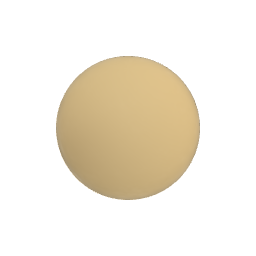
Scene (Autodesk Fusion 360 archive; units mm, degrees)
design "ball"
Autodesk Fusion 360 part; units mm, degrees
sphere "PrimitivaSfera1" add diameter 200 placed x (1, 0, 0) y (0, 1, 0) z (0, 0, 1) at (0, 0, 0)
component "Component" placed x (1, 0, 0) y (0, 1, 0) z (0, 0, 1) at (0, 0, 0)

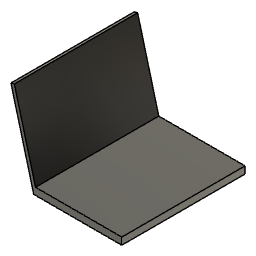
design "laptop"
Autodesk Fusion 360 part; units mm, degrees
sketch "Schizzo1" plane through (0, 0, 0) normal (0, 1, 0) x (1, 0, 0)
  line L0 (0, 0) -> (-64.7048, -241.4815)
  line L1 (-64.7048, -241.4815) -> (-55.0455, -244.0696)
  line L2 (-55.0455, -244.0696) -> (4.9938, -20)
  line L3 (4.9938, -20) -> (250, -20)
  line L4 (250, -20) -> (250, 0)
  line L5 (250, 0) -> (0, 0)
  dimension "d1" = 75
  dimension "d2" = 250
  dimension "d3" = 250
  dimension "d4" = 20
  dimension "d5" = 10
  constraint coincident L0.start L5.end
  constraint perpendicular L0 L1
  constraint perpendicular L1 L2
  constraint horizontal L3
  constraint perpendicular L3 L4
  constraint horizontal L5
  measures "d1" angle of L0 L5
  measures "d2" distance of L0.start L4.end
  measures "d3" distance of L0.start L0.end
  measures "d4" distance of L3.end L4.end
  measures "d5" distance of L0.end L1.end
extrude "Estrusione1" add sketch "Schizzo1" along normal blind 350
component "Component" placed x (1, 0, 0) y (0, 1, 0) z (0, 0, 1) at (0, 0, 0)

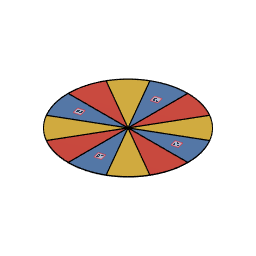
design "paracadute"
Autodesk Fusion 360 part; units mm, degrees
sketch "Schizzo1" plane through (0, 0, 0) normal (0, 0, 1) x (1, 0, 0)
  circle A0 centre (0, 0) radius 1500
  line L0 (0, 0) -> (0, 1500)
  line L1 (0, 0) -> (-750, 1299.0381)
  line L2 (0, 0) -> (-1299.0381, 750)
  line L3 (0, 0) -> (-1500, 0)
  line L4 (0, 0) -> (-1299.0381, -750)
  line L5 (0, 0) -> (-750, -1299.0381)
  line L6 (0, 0) -> (0, -1500)
  line L7 (0, 0) -> (750, -1299.0381)
  line L8 (0, 0) -> (1299.0381, -750)
  line L9 (0, 0) -> (1500, 0)
  line L10 (0, 0) -> (1299.0381, 750)
  line L11 (0, 0) -> (750, 1299.0381)
  dimension "d1" = 3000
  dimension "d3" = 360
  constraint coincident A0.centre L0.start
  constraint coincident A0 L0.end
  constraint vertical L0
  measures "d1" diameter of A0
extrude "Estrusione1" add sketch "Schizzo1" along normal blind 10 contours A0 L0 L11 makes body 1
pattern_circular "Serie C1" count 12 over 360 about axis through (0, 0, 1.75) along (0, 0, 1) of bodies 1 makes body 2 at (-441.3417, 894.9525, 0) makes body 3 at (-829.6894, 554.3807, 0) makes body 4 at (-995.7224, 65.2631, 0) makes body 5 at (-894.9525, -441.3417, 0) makes body 6 at (-554.3807, -829.6894, 0) makes body 7 at (-65.2631, -995.7224, 0) makes body 8 at (441.3417, -894.9525, 0) makes body 9 at (829.6894, -554.3807, 0) makes body 10 at (995.7224, -65.2631, 0) makes body 11 at (894.9525, 441.3417, 0) makes body 12 at (554.3807, 829.6894, 0)
sketch "Schizzo2" plane through (0, 0, 10) normal (0, 0, 1) x (-1, 0, 0)
  line L0 (0, 0) -> (0, -1500)
  arc A0 (0, -1500) -> (750, -1299.0381) centre (0, 0) ccw
  line L1 (750, -1299.0381) -> (0, 0)
  line L2 (388.2286, -1448.8887) -> (0, 0) construction
  line L3 (205.786, -1057.7817) -> (350.6749, -1018.9588)
  line L4 (350.6749, -1018.9588) -> (311.8521, -874.07)
  line L5 (311.8521, -874.07) -> (166.9632, -912.8928)
  line L6 (166.9632, -912.8928) -> (205.786, -1057.7817)
  line L7 (205.786, -1057.7817) -> (311.8521, -874.07) construction
  line L8 (350.6749, -1018.9588) -> (166.9632, -912.8928) construction
  line L9 (874.07, 311.8521) -> (912.8928, 166.9632)
  line L10 (1018.9588, 350.6749) -> (874.07, 311.8521)
  line L11 (1057.7817, 205.786) -> (1018.9588, 350.6749)
  line L12 (912.8928, 166.9632) -> (1057.7817, 205.786)
  line L13 (-311.8521, 874.07) -> (-166.9632, 912.8928)
  line L14 (-350.6749, 1018.9588) -> (-311.8521, 874.07)
  line L15 (-205.786, 1057.7817) -> (-350.6749, 1018.9588)
  line L16 (-166.9632, 912.8928) -> (-205.786, 1057.7817)
  line L17 (-874.07, -311.8521) -> (-912.8928, -166.9632)
  line L18 (-1018.9588, -350.6749) -> (-874.07, -311.8521)
  line L19 (-1057.7817, -205.786) -> (-1018.9588, -350.6749)
  line L20 (-912.8928, -166.9632) -> (-1057.7817, -205.786)
  point P0 (258.819, -965.9258)
  dimension "d8" = 500
  dimension "d9" = 150
  dimension "d10" = 150
  dimension "d12" = 360
  constraint midpoint A0 L2.start
  constraint coincident L0.start A0.centre
  constraint perpendicular L3 L4
  constraint parallel L3 L5
  constraint parallel L4 L6
  constraint coincident L7 P0
  constraint coincident L8 P0
  constraint coincident L2 P0
  constraint parallel L2 L6
  measures "d8" distance of L2.start P0
  measures "d9" distance of L3.start L3.end
  measures "d10" distance of L3.start L5.end
component "Component" placed x (1, 0, 0) y (0, 1, 0) z (0, 0, 1) at (0, 0, 0)

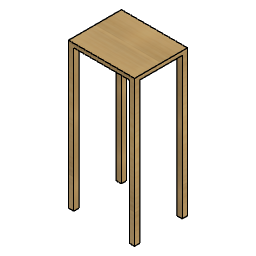
design "table"
Autodesk Fusion 360 part; units mm, degrees
box "PrimitivaParallelepipedo1" add length 400 width 500 height 30 placed x (0, 1, 0) y (-1, 0, 0) z (0, 0, 1) at (500, 0, 0)
sketch "Schizzo2" plane through (0, 0, 0) normal (0, 0, -1) x (1, 0, 0)
  line L0 (0, -400) -> (500, -400)
  line L1 (500, -400) -> (500, 0)
  line L2 (500, 0) -> (0, 0)
  line L3 (0, 0) -> (0, -400)
  line L4 (0, 0) -> (40, 0)
  line L5 (40, 0) -> (40, -40)
  line L6 (40, -40) -> (0, -40)
  line L7 (0, -40) -> (0, 0)
  line L8 (500, 0) -> (460, 0)
  line L9 (460, 0) -> (460, -40)
  line L10 (460, -40) -> (500, -40)
  line L11 (500, -40) -> (500, 0)
  line L12 (500, -400) -> (460, -400)
  line L13 (460, -400) -> (460, -360)
  line L14 (460, -360) -> (500, -360)
  line L15 (500, -360) -> (500, -400)
  line L16 (0, -400) -> (40, -400)
  line L17 (40, -400) -> (40, -360)
  line L18 (40, -360) -> (0, -360)
  line L19 (0, -360) -> (0, -400)
  dimension "d6" = 40
  dimension "d7" = 40
  dimension "d8" = 40
  dimension "d9" = 40
  constraint horizontal L4
  constraint vertical L5
  constraint horizontal L6
  constraint vertical L7
  constraint coincident L2.end L3.start
  constraint horizontal L8
  constraint vertical L9
  constraint horizontal L10
  constraint vertical L11
  constraint coincident L1.end L2.start
  constraint horizontal L12
  constraint vertical L13
  constraint horizontal L14
  constraint vertical L15
  constraint coincident L0.end L1.start
  constraint horizontal L16
  constraint vertical L17
  constraint horizontal L18
  constraint vertical L19
  constraint coincident L0.start L3.end
  constraint equal L10 L14
  constraint equal L13 L14
  constraint equal L17 L18
  constraint equal L6 L17
  measures "d6" distance of L2.end L4.end
  measures "d7" distance of L2.end L6.end
  measures "d8" distance of L1.end L8.end
  measures "d9" distance of L1.end L10.end
extrude "Estrusione1" add sketch "Schizzo2" along normal blind 1070 contours L0 L3 L16 L17 L18 L19 | L0 L1 L12 L13 L14 L15 | L2 L3 L4 L5 L6 L7 | L1 L2 L8 L9 L10 L11
component "Component" placed x (1, 0, 0) y (0, 1, 0) z (0, 0, 1) at (0, 0, 0)

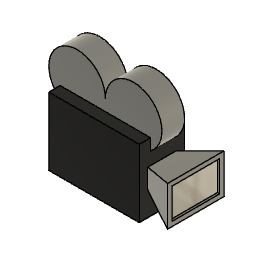
design "camera"
Autodesk Fusion 360 part; units mm, degrees
box "PrimitivaParallelepipedo1" add length 200 width 400 height 300 placed x (0, 1, 0) y (-1, 0, 0) z (0, 0, 1) at (400, 0, 0)
ref_plane "Piano di lavoro1" through (200, 100, 150) normal (0, -1, 0) x (0, 0, 1)
sketch "Schizzo2" plane through (0, 100, 0) normal (0, -1, 0) x (-1, 0, 0)
  line L0 (-400, -300) -> (-400, 0)
  line L1 (-400, 0) -> (0, 0)
  line L2 (0, 0) -> (0, -300)
  line L3 (0, -300) -> (-400, -300)
  line L4 (-325, -350) -> (-75, -350)
  line L5 (-200, -350) -> (-200, -300)
  circle A0 centre (-325, -350) radius 125
  circle A1 centre (-75, -350) radius 125
  line L6 (-325, -225) -> (-75, -225)
  dimension "d6" = 50
  dimension "d7" = 250
  constraint horizontal L4
  constraint midpoint L4 L5.start
  constraint midpoint L3 L5.end
  constraint perpendicular L3 L5
  constraint coincident L4.start A0.centre
  constraint coincident L5.start A0
  constraint coincident L4.end A1.centre
  constraint coincident L5.start A1
  constraint coincident A0 L6.start
  constraint coincident A1 L6.end
  constraint tangent A1 L6
  constraint tangent A0 L6
  measures "d6" distance of L3 L4
  measures "d7" distance of L4.start L4.end
extrude "Estrusione1" add sketch "Schizzo2" along normal mid plane 100 contours L0 L3 A0 | L3 L5 A0 | L2 L3 A1 | L3 L5 A1 picked at (-284.0328, -383.892) picked at (-121.967, -374.8835)
ref_plane "Piano di lavoro2" through (550, 100, 150) normal (1, 0, 0) x (0, 0, -1)
sketch "Schizzo3" plane through (550, 0, 0) normal (1, 0, 0) x (0, 1, 0)
  line L0 (50, 250) -> (50, 300) construction
  line L1 (50, 300) -> (0, 300) construction
  line L2 (0, 300) -> (0, 0) construction
  line L3 (0, 0) -> (200, 0) construction
  line L4 (200, 0) -> (200, 300) construction
  line L5 (200, 300) -> (150, 300) construction
  line L6 (150, 300) -> (150, 250) construction
  line L7 (150, 250) -> (50, 250) construction
  line L8 (0, 300) -> (200, 0) construction
  line L9 (225, 237.5) -> (-25, 237.5)
  line L10 (-25, 237.5) -> (-25, 62.5)
  line L11 (-25, 62.5) -> (225, 62.5)
  line L12 (225, 62.5) -> (225, 237.5)
  line L13 (225, 237.5) -> (-25, 62.5) construction
  line L14 (-25, 237.5) -> (225, 62.5) construction
  point P0 (100, 150)
  dimension "d11" = 250
  dimension "d12" = 175
  constraint coincident L1.end L2.start
  constraint coincident L3.end L4.start
  constraint horizontal L9
  constraint perpendicular L9 L10
  constraint parallel L9 L11
  constraint parallel L10 L12
  constraint coincident L13 P0
  constraint coincident L14 P0
  constraint midpoint L8 P0
  measures "d11" distance of L10.end L11.end
  measures "d12" distance of L9.end L10.end
sketch "Schizzo4" plane through (400, 0, 0) normal (1, 0, 0) x (0, 1, 0)
  line L0 (50, 250) -> (50, 300)
  line L1 (50, 300) -> (0, 300)
  line L2 (0, 300) -> (0, 0)
  line L3 (0, 0) -> (200, 0)
  line L4 (200, 0) -> (200, 300)
  line L5 (200, 300) -> (150, 300)
  line L6 (150, 300) -> (150, 250)
  line L7 (150, 250) -> (50, 250)
  line L8 (200, 300) -> (0, 0) construction
  line L9 (162.5, 193.75) -> (37.5, 193.75)
  line L10 (37.5, 193.75) -> (37.5, 106.25)
  line L11 (37.5, 106.25) -> (162.5, 106.25)
  line L12 (162.5, 106.25) -> (162.5, 193.75)
  line L13 (162.5, 193.75) -> (37.5, 106.25) construction
  line L14 (37.5, 193.75) -> (162.5, 106.25) construction
  point P0 (100, 150)
  dimension "d13" = 125
  dimension "d14" = 87.5
  constraint coincident L4.end L5.start
  constraint coincident L2.end L3.start
  constraint horizontal L9
  constraint perpendicular L9 L10
  constraint parallel L9 L11
  constraint parallel L10 L12
  constraint coincident L13 P0
  constraint coincident L14 P0
  constraint midpoint L8 P0
  measures "d13" distance of L10.end L11.end
  measures "d14" distance of L9.end L10.end
loft "Loft1" add profiles "Schizzo4", "Schizzo3" section 1 contours L9 L10 L11 L12 section 2
sketch "Schizzo5" plane through (550, 0, 0) normal (1, 0, 0) x (0, 1, 0)
  line L0 (225, 62.5) -> (225, 237.5)
  line L1 (225, 237.5) -> (-25, 237.5)
  line L2 (-25, 237.5) -> (-25, 62.5)
  line L3 (-25, 62.5) -> (225, 62.5)
  line L4 (-5, 82.5) -> (205, 82.5)
  line L5 (205, 82.5) -> (205, 217.5)
  line L6 (205, 217.5) -> (-5, 217.5)
  line L7 (-5, 217.5) -> (-5, 82.5)
  dimension "d15" = -20
extrude "Estrusione2" cut sketch "Schizzo5" against normal blind 10 contours L4 L5 L6 L7
component "Component" placed x (1, 0, 0) y (0, 1, 0) z (0, 0, 1) at (0, 0, 0)
equation "d14 = ( 175 / 2 ) * 1 mm"

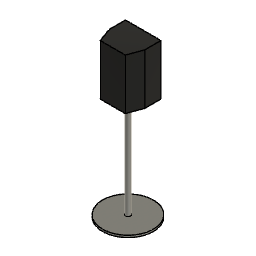
design "speaker"
Autodesk Fusion 360 part; units mm, degrees
sketch "Schizzo1" plane through (0, 0, 0) normal (0, 0, 1) x (1, 0, 0)
  circle A0 centre (0, 0) radius 250
  dimension "d1" = 500
  constraint coincident A0.centre origin
  measures "d1" diameter of A0
extrude "Estrusione1" add sketch "Schizzo1" along normal blind 20
sketch "Schizzo2" plane through (0, 0, 20) normal (0, 0, 1) x (-1, 0, 0)
  circle A0 centre (0, 0) radius 250
  circle A1 centre (0, 0) radius 25
  dimension "d4" = 50
  constraint coincident A0.centre A1.centre
  measures "d4" diameter of A1
extrude "Estrusione2" add sketch "Schizzo2" along normal blind 1000 contours A1
sketch "Schizzo3" plane through (0, 0, 1020) normal (0, 0, 1) x (-1, 0, 0)
  circle A0 centre (0, 0) radius 25
  line L0 (-175, -150) -> (175, -150)
  line L1 (175, -150) -> (175, 150)
  line L2 (175, 150) -> (-175, 150)
  line L3 (-175, 150) -> (-175, -150)
  line L4 (-175, -150) -> (175, 150) construction
  line L5 (175, -150) -> (-175, 150) construction
  line L6 (-123.697, 150) -> (-175, 9.0461)
  line L7 (123.697, 150) -> (175, 9.0461)
  dimension "d7" = 350
  dimension "d8" = 300
  dimension "d11" = 150
  dimension "d12" = 20
  dimension "d13" = 20
  constraint horizontal L0
  constraint perpendicular L0 L1
  constraint parallel L0 L2
  constraint parallel L1 L3
  constraint coincident L4 A0.centre
  constraint coincident L5 A0.centre
  constraint coincident A0.centre origin
  constraint coincident L2 L6.start
  constraint coincident L3 L6.end
  constraint coincident L2 L7.start
  constraint coincident L1 L7.end
  constraint equal L6 L7
  measures "d7" distance of L1.end L2.end
  measures "d8" distance of L0.end L1.end
  measures "d11" distance of L6.start L6.end
  measures "d12" angle of L3 L6
  measures "d13" angle of L1 L7
extrude "Estrusione3" add sketch "Schizzo3" along normal blind 500 contours A0 | L0 L1 L2 L3 L6 L7
sketch "Schizzo4" plane through (0, 150, 0) normal (0, 1, 0) x (-1, 0, 0)
  line L0 (-175, 1020) -> (175, 1020)
  line L1 (175, 1020) -> (175, 1520)
  line L2 (175, 1520) -> (-175, 1520)
  line L3 (-175, 1520) -> (-175, 1020)
  line L4 (0, 1520) -> (0, 1020) construction
  circle A0 centre (0, 1420) radius 60
  circle A1 centre (0, 1180) radius 125
  dimension "d14" = 120
  dimension "d15" = 250
  dimension "d16" = 100
  dimension "d17" = 160
  constraint midpoint L2 L4.start
  constraint midpoint L0 L4.end
  constraint coincident L4 A0.centre
  constraint coincident L4 A1.centre
  measures "d14" diameter of A0
  measures "d15" diameter of A1
  measures "d16" distance of L2 A0.centre
  measures "d17" distance of L0 A1.centre
extrude "Estrusione4" cut sketch "Schizzo4" against normal blind 20 contours A0 | A1
component "Component" placed x (1, 0, 0) y (0, 1, 0) z (0, 0, 1) at (0, 0, 0)
